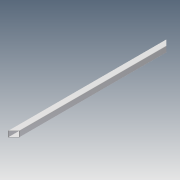
# Autodesk Inventor part: frame open end rail
Saved by Autodesk Inventor 2014 (Build 180170000, 170)
## iProperties
Created: 2016-01-12
Part Number: frame open end rail
Material: Steel, Mild
Document SubType Name: Modeling
Designer: Paul
Density: 7.86 g/cm^3
Appearance: Steel
Mass: 776.801 g
Surface Area: 1239.45 cm^2
Volume: 98.8297 cm^3
Author: Paul
Autodesk Inventor part; units mm, degrees
ref_plane "YZ Plane" through (0, 0, 0) normal (1, 0, 0) x (0, 1, 0)
ref_plane "XZ Plane" through (0, 0, 0) normal (0, 1, 0) x (-1, 0, 0)
ref_plane "XY Plane" through (0, 0, 0) normal (0, 0, 1) x (1, 0, 0)
sketch "Sketch1" plane through (0, 0, 0) normal (0, 0, 1) x (1, 0, 0)
  line L0 (1.778, 0) -> (23.622, 0)
  line L1 (25.4, 1.778) -> (25.4, 23.622)
  line L2 (23.622, 25.4) -> (1.778, 25.4)
  line L3 (0, 23.622) -> (0, 1.778)
  arc A0 (1.778, 25.4) -> (0, 23.622) centre (1.778, 23.622) ccw
  arc A1 (25.4, 23.622) -> (23.622, 25.4) centre (23.622, 23.622) ccw
  arc A2 (23.622, 0) -> (25.4, 1.778) centre (23.622, 1.778) ccw
  arc A3 (0, 1.778) -> (1.778, 0) centre (1.778, 1.778) ccw
  line L4 (23.7998, 23.622) -> (23.7998, 1.778)
  arc A4 (23.622, 1.6002) -> (23.7998, 1.778) centre (23.622, 1.778) ccw
  line L5 (23.622, 1.6002) -> (1.778, 1.6002)
  arc A5 (1.6002, 1.778) -> (1.778, 1.6002) centre (1.778, 1.778) ccw
  line L6 (1.6002, 1.778) -> (1.6002, 23.622)
  arc A6 (1.778, 23.7998) -> (1.6002, 23.622) centre (1.778, 23.622) ccw
  line L7 (1.778, 23.7998) -> (23.622, 23.7998)
  arc A7 (23.7998, 23.622) -> (23.622, 23.7998) centre (23.622, 23.622) ccw
  point P0 (0, 0)
  point P1 (25.4, 25.4)
  point P2 (25.4, 0)
  point P3 (0, 25.4)
  dimension "d0" = 25.4
  dimension "d1" = 25.4
  dimension "d2" = 1.778
  dimension "d3" = 1.6002
  constraints: 16 end point, 16 point on circle, 8 centre point, 8 point on line, 8 tangent, 4 parallel, 3 equal radius, 2 perpendicular, 1 horizontal, 7 other
  measures "d0" distance of point (0, 25.4) point (25.4, 25.4)
  measures "d1" distance of point (25.4, 25.4) point (25.4, 0)
  measures "d2" radius of A0
  measures "d3" distance between parallel lines of L4 L1
extrude "Extrusion1" add sketch "Sketch1" along normal blind 685.8
sketch "Sketch2" plane through (1.778, 25.4, 0) normal (0, 1, 0) x (1, 0, 0)
  line L0 (-1.778, 0) -> (-1.778, -685.8) projected
  line L1 (23.622, 0) -> (23.622, -685.8) projected
  line L2 (-1.778, 0) -> (23.622, -25.4)
  line L3 (-1.778, 0) -> (74.422, 0) construction
  line L4 (23.622, -25.4) -> (23.622, 0)
  line L5 (-1.778, 0) -> (23.622, 0)
  line L6 (-1.778, -685.8) -> (23.622, -660.4)
  line L7 (-1.778, -685.8) -> (74.422, -685.8) construction
  line L8 (-1.778, -685.8) -> (23.622, -685.8)
  line L9 (23.622, -660.4) -> (23.622, -685.8)
  dimension "d7" = 45
  dimension "d9" = 45
  constraints: 16 end point, 3 perpendicular, 3 point on line, 2 collinear, 2 horizontal
  measures "d7" angle of L2 L3
  measures "d9" angle of L7 L6
extrude "Extrusion2" cut sketch "Sketch2" against normal blind 25.4 contours L5 L1 L2 | L6 L1 L8
body "Solid1"
